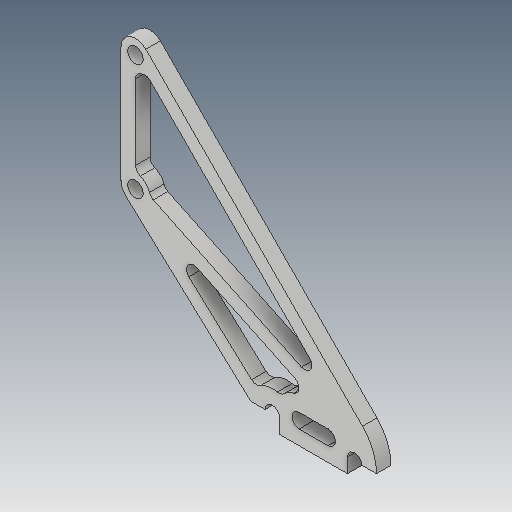
# Autodesk Inventor part: Tens1
Saved by Autodesk Inventor 2019.4 (Build 234330000, 330)
## iProperties
Created: 2019-06-15
Part Number: Tens1
Material: Generic
Document SubType Name: Modeling
Designer: AzLIer
Density: 1 g/cm^3
Appearance: Default
Mass: 2.04362 g
Surface Area: 25.1733 cm^2
Volume: 2.04362 cm^3
Author: AzLIer
Autodesk Inventor part; units mm, degrees
ref_plane "YZ Plane" through (0, 0, 0) normal (1, 0, 0) x (0, 1, 0)
ref_plane "XZ Plane" through (0, 0, 0) normal (0, 1, 0) x (-1, 0, 0)
ref_plane "XY Plane" through (0, 0, 0) normal (0, 0, 1) x (1, 0, 0)
sketch "スケッチ1" plane through (0, 0, 0) normal (0, 0, 1) x (1, 0, 0)
  circle A0 centre (0, 0) radius 1.6
  arc A1 (2.1289, 2.1137) -> (-3, 0) centre (0, 0) ccw
  line L0 (43.813, -50.0351) -> (43.8106, -53.0351) projected
  line L1 (29.813, -50.0239) -> (29.8106, -53.0239) projected
  line L2 (46.9094, -42.9894) -> (2.1289, 2.1137)
  arc A2 (49.813, -50.0351) -> (46.9094, -42.9894) centre (39.813, -50.0351) ccw
  line L3 (49.813, -50.0351) -> (49.813, -50.0351)
  line L4 (49.813, -50.0351) -> (46.813, -50.0351)
  arc A3 (46.813, -50.0351) -> (43.813, -50.0351) centre (45.313, -50.0363) ccw
  line L5 (43.8106, -53.0351) -> (29.8106, -53.0239)
  arc A4 (29.813, -50.0239) -> (26.8131, -50.0351) centre (28.313, -50.0227) ccw
  line L6 (39.8106, -48.5351) -> (33.8106, -48.5351) construction
  line L7 (39.8106, -47.0351) -> (33.8106, -47.0351)
  line L8 (33.8106, -50.0351) -> (39.8106, -50.0351)
  arc A5 (39.8106, -50.0351) -> (39.8106, -47.0351) centre (39.8106, -48.5351) ccw
  arc A6 (33.8106, -47.0351) -> (33.8106, -50.0351) centre (33.8106, -48.5351) ccw
  line L9 (23.8131, -50.0351) -> (26.8131, -50.0351)
  circle A7 centre (0, -24) radius 1.6
  arc A8 (-3, -24) -> (-2.0335, -26.2056) centre (0, -24) ccw
  line L10 (-3, -24) -> (-3, 0)
  line L11 (-2.0335, -26.2056) -> (23.8131, -50.0351)
  point P0 (36.8106, -53.0295)
  point P1 (36.8106, -48.5351)
  point P2 (36.8106, -50.0351)
  dimension "d0" = 3.2
  dimension "d1" = 6
  dimension "d4" = 1.5
  dimension "d5" = 3
  dimension "d8" = 6
  dimension "d9" = 1.5
  dimension "d10" = 3
  dimension "d13" = 10
  dimension "d14" = 3.2
  dimension "d15" = 24
  constraints: 22 end point, 14 point on circle, 12 tangent, 9 centre point, 3 coincident, 3 midpoint, 3 point on line, 2 equal radius, 2 vertical alignment, 1 collinear, 1 horizontal, 1 line through centre, 1 parallel, 1 perpendicular, 1 vertical
  measures "d0" diameter of A0
  measures "d1" diameter of A1
  measures "d4" radius of A3
  measures "d5" distance of L4.end L3.end
  measures "d8" distance of L6.start L6.end
  measures "d9" radius of A5
  measures "d10" distance of L9.start L9.end
  measures "d13" radius of A2
  measures "d14" diameter of A7
  measures "d15" distance of A7.centre point (0, 0)
extrude "押し出し1" add sketch "スケッチ1" along normal blind 3
sketch "スケッチ2" plane through (0, 0, 3) normal (0, 0, 1) x (1, 0, 0)
  arc A0 (39.8106, -50.0351) -> (39.8106, -47.0351) centre (39.8106, -48.5351) ccw projected
  line L0 (39.8106, -50.0351) -> (33.8106, -50.0351) projected
  arc A1 (33.8106, -47.0351) -> (33.8106, -50.0351) centre (33.8106, -48.5351) ccw projected
  line L1 (33.8106, -47.0351) -> (39.8106, -47.0351) projected
  circle A2 centre (0, -24) radius 1.6 projected
  circle A3 centre (0, 0) radius 1.6 projected
  arc A4 (46.813, -50.0351) -> (43.813, -50.0351) centre (45.313, -50.0363) ccw projected
  line L2 (46.813, -50.0351) -> (49.813, -50.0351) projected
  arc A5 (49.813, -50.0351) -> (46.9094, -42.9894) centre (39.813, -50.0351) ccw projected
  line L3 (46.9094, -42.9894) -> (2.1289, 2.1137) projected
  arc A6 (2.1289, 2.1137) -> (-3, 0) centre (0, 0) ccw projected
  line L4 (-3, 0) -> (-3, -24) projected
  arc A7 (-3, -24) -> (-2.0335, -26.2056) centre (0, -24) ccw projected
  line L5 (-2.0335, -26.2056) -> (23.8131, -50.0351) projected
  line L6 (23.8131, -50.0351) -> (26.8131, -50.0351) projected
  arc A8 (29.813, -50.0239) -> (26.8131, -50.0351) centre (28.313, -50.0227) ccw projected
  line L7 (29.813, -50.0239) -> (29.8106, -53.0239) projected
  line L8 (29.8106, -53.0239) -> (43.8106, -53.0351) projected
  line L9 (43.8106, -53.0351) -> (43.813, -50.0351) projected
  arc A9 (45.1777, -45.5383) -> (44.7805, -45.1031) centre (39.813, -50.0351) ccw
  arc A10 (45.1777, -45.5383) -> (40.813, -50.0327) centre (45.313, -50.0363) ccw
  line L10 (40.813, -50.0327) -> (32.813, -50.0263)
  arc A11 (39.8106, -53.0351) -> (43.4781, -45.9274) centre (39.8106, -48.5351) ccw
  line L11 (39.8106, -53.0351) -> (33.8106, -53.0351)
  line L12 (33.8106, -44.0351) -> (38.5389, -44.0351)
  line L13 (0, -24) -> (45.1777, -45.5383) construction
  arc A12 (0, -22.5) -> (-0.6455, -25.354) centre (0, -24) ccw
  arc A13 (44.5321, -46.8923) -> (45.8232, -44.1843) centre (45.1777, -45.5383) ccw
  line L14 (43.0134, -46.1682) -> (44.5321, -46.8923)
  arc A14 (32.813, -50.0263) -> (32.3777, -48.0917) centre (28.313, -50.0227) ccw
  arc A15 (30.1517, -45.9155) -> (24.9646, -47.0163) centre (28.313, -50.0227) ccw
  arc A16 (33.8106, -44.0351) -> (30.1517, -45.9155) centre (33.8106, -48.5351) ccw
  arc A17 (29.3269, -48.9172) -> (33.8106, -53.0351) centre (33.8106, -48.5351) ccw
  line L15 (0, 0) -> (1.1273, -1.1354)
  line L16 (2.1137, -2.1289) -> (42.1113, -42.4147)
  line L17 (0, -1.6) -> (0, 0)
  arc A18 (2.1289, 2.1137) -> (-3, 0) centre (0, 0) ccw
  arc A19 (0, -3) -> (2.1137, -2.1289) centre (0, 0) ccw
  line L18 (-0.6455, -25.354) -> (1.6997, -26.4721)
  line L19 (3.7325, -27.4412) -> (38.5389, -44.0351)
  line L20 (24.9646, -47.0163) -> (3.7325, -27.4412)
  line L21 (2.2056, -26.0335) -> (0, -24)
  line L22 (42.1113, -42.4147) -> (2.9907, -23.7641)
  line L23 (1.1481, -22.8856) -> (0.6455, -22.646)
  line L24 (0, -24) -> (0, -22.4)
  line L25 (0, -21) -> (0, -3)
  arc A20 (2.9907, -23.7641) -> (0, -21) centre (0, -24) ccw
  arc A21 (-3, -24) -> (2.2056, -26.0335) centre (0, -24) ccw
  point P0 (22.5888, -34.7692)
  dimension "d17" = 3
  dimension "d18" = 3
  constraints: 37 end point, 35 point on circle, 13 centre point, 10 tangent, 6 parallel, 2 coincident, 1 midpoint, 1 point on line, 2 other
  measures "d17" distance between parallel lines of L1 L12
  measures "d18" diameter of A13
extrude "押し出し2" cut sketch "スケッチ2" against normal blind 3 contours A16 A15 L20 L19 L12 | L16 L22 A20 L25 A19
fillet "フィレット1" radius 1.5 9 edges at (24.9646, -47.0163, 1.5) (30.1517, -45.9155, 1.5) (38.5389, -44.0351, 1.5) (3.7325, -27.4412, 1.5) (0, -21, 1.5) (2.9907, -23.7641, 1.5) (0, -3, 1.5) (2.1137, -2.1289, 1.5) (42.1113, -42.4147, 1.5)
